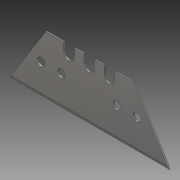
# Autodesk Inventor part: Rasierklinge
Saved by Autodesk Inventor 2019.4 (Build 234330000, 330)
## iProperties
Part Number: Rasierklinge
Material: Stahl, weich
Document SubType Name: Modeling
Designer: rYan
Mass: 2.65476 g
Surface Area: 14.6846 cm^2
Volume: 0.338186 cm^3
Density: 7.85 g/cm^3
Appearance: Halbpoliert
Author: rYan
Autodesk Inventor part; units mm, degrees
ref_plane "YZ Plane" through (0, 0, 0) normal (1, 0, 0) x (0, 1, 0)
ref_plane "XZ Plane" through (0, 0, 0) normal (0, 1, 0) x (-1, 0, 0)
ref_plane "XY Plane" through (0, 0, 0) normal (0, 0, 1) x (1, 0, 0)
sketch "Skizze1" plane through (0, 0, 0) normal (0, 1, 0) x (-1, 0, 0)
  line L0 (26.1, 0) -> (14.2, 19)
  line L1 (-14.2, 19) -> (-26.1, 0)
  line L2 (-26.1, 0) -> (26.1, 0)
  line L3 (0, -3.8) -> (0, 22.8) projected
  line L4 (1.75, 19) -> (1.75, 16.35)
  line L5 (-1.75, 19) -> (-1.75, 16.35)
  line L6 (-4.85, 19) -> (-4.85, 16.35)
  line L7 (-8.35, 19) -> (-8.35, 16.35)
  line L8 (4.85, 19) -> (4.85, 16.35)
  line L9 (8.35, 19) -> (8.35, 16.35)
  arc A0 (4.85, 16.35) -> (8.35, 16.35) centre (6.6, 16.35) ccw
  arc A1 (-1.75, 16.35) -> (1.75, 16.35) centre (0, 16.35) ccw
  arc A2 (-8.35, 16.35) -> (-4.85, 16.35) centre (-6.6, 16.35) ccw
  line L10 (-1.75, 19) -> (-4.85, 19)
  line L11 (-8.35, 19) -> (-14.2, 19)
  line L12 (14.2, 19) -> (8.35, 19)
  line L13 (4.85, 19) -> (1.75, 19)
  line L14 (6.6, 16.35) -> (-6.6, 16.35) construction
  circle A3 centre (15.7, 9.75) radius 1.35
  circle A4 centre (9.1, 9.75) radius 1.35
  circle A5 centre (-9.1, 9.75) radius 1.35
  circle A6 centre (-15.7, 9.75) radius 1.35
  line L15 (15.7, 9.75) -> (-15.7, 9.75) construction
  point P0 (0, 0)
  dimension "d1" = 52.2
  dimension "d2" = 28.4
  dimension "d3" = 3.5
  dimension "d4" = 19
  dimension "d5" = 2.65
  dimension "d6" = 3.5
  dimension "d7" = 3.1
  dimension "d8" = 2.7
  dimension "d9" = 9.25
  dimension "d10" = 6.6
  dimension "d11" = 18.2
  constraints: 30 end point, 7 centre point, 6 horizontal, 6 point on circle, 6 tangent, 6 vertical, 4 parallel, 3 collinear, 3 equal radius, 2 midpoint, 2 point on line, 6 other
  measures "d1" distance of L1.end L0.start
  measures "d2" distance of L0.end L1.start
  measures "d3" distance between parallel lines of L5 L4
  measures "d4" distance between parallel lines of L2 L11
  measures "d5" distance of L4.start L4.end
  measures "d6" distance between parallel lines of L8 L9
  measures "d7" distance of L5.start L6.start
  measures "d8" diameter of A3
  measures "d9" distance between parallel lines of L15 L12
  measures "d10" distance of A4.centre L15.start
  measures "d11" distance of A5.centre A4.centre
extrude "Extrusion1" add sketch "Skizze1" along normal blind 0.5
chamfer "Fase1" distance 0.25 angle 75 4 edges at (13.05, 0, 0) (-13.05, 0, 0) (13.05, 0.5, 0) (-13.05, 0.5, 0) measured on face at (17.4, 0.1667, 0) measured on face at (-8.7, 0.1667, 0)
equation "\"d6\" = d3"
